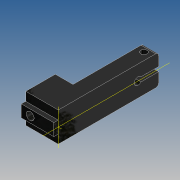
# Autodesk Inventor part: P116SupportFibre
Saved by Autodesk Inventor 2017 (Build 210142000, 142)
## iProperties
Created: 2016-12-15
Part Number: P116SupportFibre
Material: ABS
Document SubType Name: Modeling
Designer: serge.amoos
Density: 1.06 g/cm^3
Appearance: Smooth - Black
Author: serge.amoos
Autodesk Inventor part; units mm, degrees
ref_plane "YZ Plane" through (0, 0, 0) normal (1, 0, 0) x (0, 1, 0)
ref_plane "XZ Plane" through (0, 0, 0) normal (0, 1, 0) x (-1, 0, 0)
ref_plane "XY Plane" through (0, 0, 0) normal (0, 0, 1) x (1, 0, 0)
sketch "Sketch1" plane through (0, 0, 0) normal (0, 0, 1) x (1, 0, 0)
  line L0 (-26.4, 0) -> (4.4, 0) construction
  line L1 (0, -28.2297) -> (0, 100.056) construction
  line L2 (0, 0) -> (-22, 0)
  line L3 (-22, 0) -> (-22, 20)
  line L4 (-22, 20) -> (-10, 20)
  line L5 (-10, 20) -> (-10, 68)
  line L6 (-10, 68) -> (0, 68)
  line L7 (0, 68) -> (0, 0)
  dimension "d0" = 68
  dimension "d1" = 10
  dimension "d2" = 22
  dimension "d3" = 20
  constraints: 12 end point, 4 perpendicular, 2 point on line, 1 vertical
  measures "d0" distance between parallel lines of L0 L6
  measures "d1" distance between parallel lines of L7 L5
  measures "d2" distance between parallel lines of L1 L3
  measures "d3" distance between parallel lines of L0 L4
extrude "Extrusion1" add sketch "Sketch1" along normal mid plane 20
sketch "Sketch2" plane through (-22, 0, 10) normal (0, -1, 0) x (1, 0, 0)
  line L0 (-4.4, -10) -> (26.4, -10) construction
  line L1 (22, -24) -> (22, 4) construction
  line L2 (0, 0) -> (0, -20) construction
  line L3 (0, -5.9) -> (22, -5.9)
  line L4 (22, -5.9) -> (22, -14.1)
  line L5 (22, -14.1) -> (0, -14.1)
  line L6 (0, -14.1) -> (0, -5.9)
  point P0 (22, -10)
  point P1 (22, -10)
  dimension "d6" = 8.2
  constraints: 8 end point, 3 point on line, 2 parallel, 1 horizontal, 1 midpoint, 1 perpendicular
  measures "d6" distance between parallel lines of L5 L3
extrude "Extrusion2" add sketch "Sketch2" along normal blind 3
sketch "Sketch4" plane through (-22, 20, 10) normal (0, 1, 0) x (1, 0, 0)
  line L0 (-4.4, 10) -> (26.4, 10) projected
  line L1 (22, 24) -> (22, -4) projected
  point P0 (22, 10)
  point P1 (6, 10)
  dimension "d18" = 16
  constraints: 1 point on line
  measures "d18" distance from line of L1 point (6, 10)
hole "Hole2" at (-16, 20, 0) direction (0, -1, 0) diameter 5.3 end through all
sketch "Esquisse5" plane through (-10, 20, -10) normal (-1, 0, 0) x (0, 0, 1)
  line L0 (10, -33.1749) -> (10, 52.2673)
  line L1 (5.9, -20) -> (0, -20) projected
  point P0 (10, -20)
  point P1 (10, 34)
  dimension "d28" = 54
  constraints: 2 end point, 1 point on line, 1 vertical
  measures "d28" distance from line of L1 point (10, 34)
hole "Perçage3" at (-10, 54, 0) direction (1, 0, 0) diameter 5 end through all
fillet "Congé2" radius 2 1 edges at (-5, 68, -10)
fillet "Congé3" radius 2 1 edges at (-5, 68, 10)
sketch "Esquisse6" plane through (-10, 20, -10) normal (-1, 0, 0) x (0, 0, 1)
  line L0 (10, -28.7649) -> (10, 59.9082)
  line L1 (5.9, -20) -> (0, -20) projected
  point P0 (10, -20)
  point P1 (10, 34)
  dimension "d38" = 54
  constraints: 2 end point, 1 point on line, 1 vertical
  measures "d38" distance from line of L1 point (10, 34)
hole "Perçage4" at (-10, 54, 0) direction (1, 0, 0) diameter 10.5 depth 6
sketch "Esquisse8" plane through (-10, 20, -10) normal (-1, 0, 0) x (0, 0, 1)
  line L0 (10, -28.9396) -> (10, 64.2926)
  line L1 (10, 34) -> (8.5, 34)
  line L2 (8.5, 34) -> (8.5, 50.8033)
  line L3 (8.5, 50.8033) -> (10, 50.8033)
  line L4 (5.9, -20) -> (0, -20) projected
  line L5 (20, 46) -> (20, 0) projected
  line L6 (10, 34) -> (10, 50.8033)
  point P0 (10, -20)
  dimension "d50" = 54
  dimension "d51" = 3
  dimension "d52" = 10
  dimension "d53" = 16.8033
  dimension "d54" = 8.9396
  dimension "d55" = 93.2322
  constraints: 10 end point, 2 perpendicular, 2 point on line, 1 collinear, 1 parallel, 1 vertical
  measures "d50" distance between parallel lines of L4 L1
  measures "d51" diameter of L2 L0
  measures "d52" distance between parallel lines of L5 L0
  measures "d53" distance between parallel lines of L3 L1
  measures "d54" distance of point (10, -20) L0.start
  measures "d55" distance of L0.start L0.end
extrude "Extrusion3" cut sketch "Esquisse8" against normal through all
mirror "Symétrie1" about plane through (-10, 70.8033, 0) normal (0, 0, -1) of "Extrusion3"
sketch "Esquisse9" plane through (0, 0, 10) normal (0, 0, 1) x (1, 0, 0)
  line L0 (-10, 66) -> (-10, 20) projected
  line L1 (-22, 0) -> (0, 0) projected
  point P0 (-5, 63)
  dimension "d58" = 5
  dimension "d59" = 63
  measures "d58" distance from line of L0 point (-5, 63)
  measures "d59" distance from line of L1 point (-5, 63)
hole "Perçage5" at (-5, 63, 10) direction (0, 0, -1) diameter 4.2 end through all
body "Solid1"
